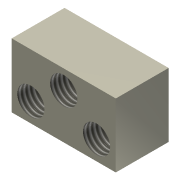
# Autodesk Inventor part: Solenoid Base 1764
Saved by Autodesk Inventor 2011 (Build 150239000, 239)
## iProperties
Created: 2010-02-15
Part Number: Solenoid Base 1764
Document SubType Name: Modeling
Designer: jgehrig
Density: 1 g/cm^3
Author: jgehrig
Autodesk Inventor part; units mm, degrees
ref_plane "YZ Plane" through (0, 0, 0) normal (1, 0, 0) x (0, 1, 0)
ref_plane "XZ Plane" through (0, 0, 0) normal (0, 1, 0) x (-1, 0, 0)
ref_plane "XY Plane" through (0, 0, 0) normal (0, 0, 1) x (1, 0, 0)
sketch "Sketch1" plane through (0, 0, 0) normal (0, 0, 1) x (1, 0, 0)
  line L0 (-30.2326, 17.8682) -> (11.0424, 17.8682)
  line L1 (11.0424, 17.8682) -> (11.0424, -7.5318)
  line L2 (11.0424, -7.5318) -> (-30.2326, -7.5318)
  line L3 (-30.2326, -7.5318) -> (-30.2326, 17.8682)
  point P0 (0, 0)
  dimension "d0" = 41.275
  dimension "d1" = 25.4
  constraints: 8 end point, 2 parallel, 1 horizontal, 1 perpendicular
  measures "d0" distance of L0.start L0.end
  measures "d1" distance of L2.end L0.start
extrude "Extrusion1" add sketch "Sketch1" along normal blind 20.955
sketch "Sketch2" plane through (0, 0, 20.955) normal (0, 0, 1) x (1, 0, 0)
  line L0 (11.0424, 17.8682) -> (11.0424, -7.5318) projected
  line L1 (-30.2326, 17.8682) -> (11.0424, 17.8682) projected
  line L2 (-30.2326, -7.5318) -> (-30.2326, 17.8682) projected
  line L3 (11.0424, -7.5318) -> (-30.2326, -7.5318) projected
  circle A0 centre (-9.5951, 10.2482) radius 5.3975
  circle A1 centre (-22.6126, 0.0882) radius 5.3975
  circle A2 centre (3.4224, 0.0882) radius 5.3975
  dimension "d4" = 10.795
  dimension "d5" = 7.62
  dimension "d6" = 7.62
  dimension "d7" = 7.62
  dimension "d8" = 7.62
  dimension "d9" = 7.62
  constraints: 3 centre point, 2 equal radius
  measures "d4" diameter of A0
  measures "d5" distance from line of L1 A0.centre
  measures "d6" distance from line of L3 A1.centre
  measures "d7" distance from line of L3 A2.centre
  measures "d8" distance from line of L2 A1.centre
  measures "d9" distance from line of L0 A2.centre
extrude "Extrusion2" cut sketch "Sketch2" against normal blind 9.525 contours A0 | A1 | A2
thread "Thread1" size "7/16-14 UNC" class "2B" standard "ANSI Unified Screw Threads" full length
thread "Thread2" size "7/16-14 UNC" class "2B" standard "ANSI Unified Screw Threads" full length
thread "Thread3" size "7/16-14 UNC" class "2B" standard "ANSI Unified Screw Threads" full length
sketch "Sketch3" plane through (0, 0, 0) normal (0, 0, -1) x (-1, 0, 0)
  line L0 (30.2326, -7.5318) -> (30.2326, 17.8682) projected
  circle A0 centre (0.0701, 5.1682) radius 5.3975
  circle A1 centre (19.1201, 5.1682) radius 5.3975
  point P0 (0, 0)
  dimension "d18" = 10.795
  dimension "d19" = 19.05
  dimension "d20" = 11.1125
  constraints: 2 centre point, 1 equal radius
  measures "d18" diameter of A0
  measures "d19" distance of A1.centre A0.centre
  measures "d20" distance from line of L0 A1.centre
extrude "Extrusion3" cut sketch "Sketch3" against normal blind 9.525
thread "Thread4" size "7/16-14 UNC" class "2B" standard "ANSI Unified Screw Threads" full length
thread "Thread5" size "7/16-14 UNC" class "2B" standard "ANSI Unified Screw Threads" full length
body "Solid1"
